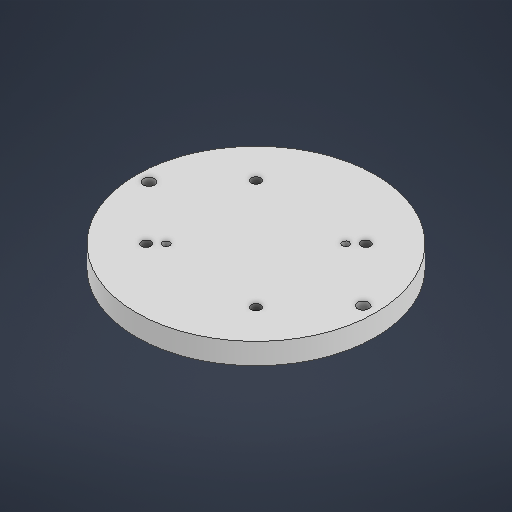
# Autodesk Inventor part: substrate plate
Saved by Autodesk Inventor 2025 (Build 290162000, 162)
## iProperties
Created: 2024-06-21
Part Number: substrate plate
Material: Generic
Document SubType Name: Modeling
Designer: mayhe
Density: 1 g/cm^3
Appearance: Default
Author: mayhe
Autodesk Inventor part; units mm, degrees
ref_plane "YZ Plane" through (0, 0, 0) normal (1, 0, 0) x (0, 1, 0)
ref_plane "XZ Plane" through (0, 0, 0) normal (0, 1, 0) x (-1, 0, 0)
ref_plane "XY Plane" through (0, 0, 0) normal (0, 0, 1) x (1, 0, 0)
sketch "Sketch1" plane through (0, 0, 0) normal (0, 1, 0) x (-1, 0, 0)
  circle A0 centre (0, 0) radius 84.75
  dimension "d0" = 169.5
  constraints: 1 centre point, 1 coincident
  measures "d0" diameter of A0
extrude "Extrusion1" add sketch "Sketch1" along normal blind 15
sketch "Sketch2" plane through (0, 0, 0) normal (0, -1, 0) x (1, 0, 0)
  circle A0 centre (0, 0) radius 76
  circle A1 centre (0, 76) radius 4
  circle A2 centre (0, -76) radius 4
  circle A3 centre (0, 76) radius 2.25
  circle A4 centre (0, -76) radius 2.25
  dimension "d3" = 152
  dimension "d4" = 8
  dimension "d5" = 8
  dimension "d6" = 4.5
  dimension "d7" = 4.5
  constraints: 5 centre point, 3 point on circle, 2 coincident
  measures "d3" diameter of A0
  measures "d4" diameter of A1
  measures "d5" diameter of A2
  measures "d6" diameter of A3
  measures "d7" diameter of A4
extrude "Extrusion2" cut sketch "Sketch2" against normal through all contours A3 A0 | A0 A3 | A4 A0 | A0 A4
extrude "Extrusion3" cut sketch "Sketch2" against normal blind 12 contours A1 A0 A3 | A0 A3 A1 | A2 A0 A4 | A0 A4 A2 | A3 A0 | A0 A3 | A4 A0 | A0 A4
sketch "Sketch3" plane through (0, 0, 0) normal (0, -1, 0) x (1, 0, 0)
  circle A0 centre (0, 0) radius 84.75
  circle A1 centre (0, 0) radius 20
  circle A2 centre (0, -20) radius 4
  circle A3 centre (20, 0) radius 4
  circle A4 centre (0, 20) radius 4
  circle A5 centre (-20, 0) radius 4
  line L0 (55, 55) -> (-55, 55)
  line L1 (-55, 55) -> (-55, -55)
  line L2 (-55, -55) -> (55, -55)
  line L3 (55, -55) -> (55, 55)
  line L4 (55, 55) -> (-55, -55) construction
  line L5 (-55, 55) -> (55, -55) construction
  circle A6 centre (0, 0) radius 55
  circle A7 centre (-38.8909, -38.8909) radius 4
  circle A8 centre (38.8909, -38.8909) radius 4
  circle A9 centre (38.8909, 38.8909) radius 4
  circle A10 centre (-38.8909, 38.8909) radius 4
  dimension "d12" = 40
  dimension "d13" = 8
  dimension "d16" = 360
  dimension "d21" = 110
  dimension "d22" = 110
  dimension "d23" = 110
  dimension "d24" = 8
  dimension "d25" = 8
  dimension "d26" = 8
  dimension "d27" = 8
  constraints: 12 end point, 10 centre point, 4 point on circle, 4 point on line, 3 coincident, 2 midpoint, 2 parallel, 1 horizontal, 1 perpendicular, 1 vertical alignment, 11 other
  measures "d13" diameter of A2
  measures "d21" distance of L2.end L1.end
  measures "d22" distance of L1.end L0.end
  measures "d23" diameter of A6
  measures "d24" diameter of A7
  measures "d25" diameter of A8
  measures "d26" diameter of A9
  measures "d27" diameter of A10
hole "Hole1" at (38.8909, 0, -38.8909) at (38.8909, 0, 38.8909) at (-38.8909, 0, 38.8909) at (-38.8909, 0, -38.8909) direction (0, 1, 0) diameter 6.647 depth 12 tip angle 118 thread size "M8x1.25" class "6H" standard "ANSI Metric M Profile"
sketch "Sketch4" plane through (0, 0, 0) normal (0, -1, 0) x (1, 0, 0)
  circle A0 centre (0, 0) radius 45
  circle A1 centre (-45, 0) radius 2.5
  circle A2 centre (-41.5746, -17.2208) radius 2.5
  circle A3 centre (-31.8198, -31.8198) radius 2.5
  circle A4 centre (-17.2208, -41.5746) radius 2.5
  circle A5 centre (0, -45) radius 2.5
  circle A6 centre (17.2208, -41.5746) radius 2.5
  circle A7 centre (31.8198, -31.8198) radius 2.5
  circle A8 centre (41.5746, -17.2208) radius 2.5
  circle A9 centre (45, 0) radius 2.5
  circle A10 centre (41.5746, 17.2208) radius 2.5
  circle A11 centre (31.8198, 31.8198) radius 2.5
  circle A12 centre (17.2208, 41.5746) radius 2.5
  circle A13 centre (0, 45) radius 2.5
  circle A14 centre (-17.2208, 41.5746) radius 2.5
  circle A15 centre (-31.8198, 31.8198) radius 2.5
  circle A16 centre (-41.5746, 17.2208) radius 2.5
  dimension "d35" = 90
  dimension "d36" = 5
  dimension "d39" = 360
  constraints: 16 centre point, 1 coincident, 1 horizontal alignment, 35 other
  measures "d36" diameter of A1
hole "Hole2" at (-31.8198, 0, 31.8198) at (31.8198, 0, -31.8198) direction (0, 1, 0) diameter 5 end through all
body "Solid1"
